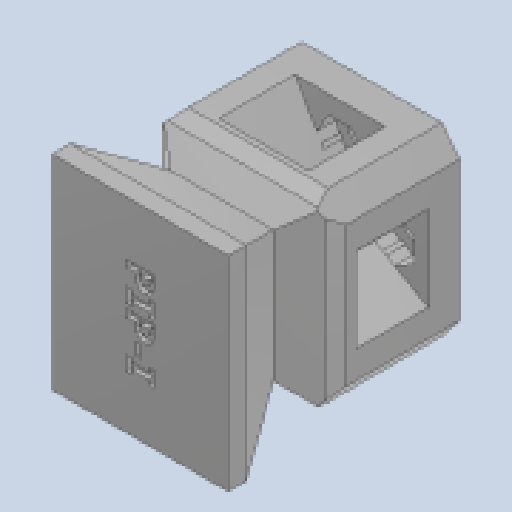
# Autodesk Inventor part: PIP-I
Saved by Autodesk Inventor 2026 (Build 300175050, 175E)
## iProperties
Created: 2025-12-11
Part Number: PIP-I
Material: Genérico
Document SubType Name: Modeling
Designer: user
Density: 1 g/cm^3
Appearance: Suave - Gris medio
Author: user
Autodesk Inventor part; units mm, degrees
ref_plane "YZ Plane" through (0, 0, 0) normal (1, 0, 0) x (0, 1, 0)
ref_plane "XZ Plane" through (0, 0, 0) normal (0, 1, 0) x (-1, 0, 0)
ref_plane "XY Plane" through (0, 0, 0) normal (0, 0, 1) x (1, 0, 0)
sketch "Boceto1" plane through (0, 0, 0) normal (0, 0, 1) x (1, 0, 0)
  line L0 (9.7, 16.5) -> (9.7, -16.5) projected
  line L1 (9.7, 16.5) -> (-9.7, 16.5) projected
  line L2 (-9.7, -16.5) -> (-9.7, 16.5) projected
  line L3 (9.7, -16.5) -> (-9.7, -16.5) projected
  circle A0 centre (8, 8) radius 0.8 construction
  circle A1 centre (-8, -8) radius 0.8 construction
  circle A2 centre (8, -8) radius 0.8 construction
  circle A3 centre (0, 0) radius 4 construction
  circle A4 centre (0, -6) radius 1.025 construction
  circle A5 centre (6, 0) radius 1.025 construction
  circle A6 centre (0, 6) radius 1.025 construction
  circle A7 centre (-6, 0) radius 1.025 construction
  circle A8 centre (-5.6569, -5.6569) radius 1.025 construction
  circle A9 centre (5.6569, -5.6569) radius 1.025 construction
  circle A10 centre (-5.6569, 5.6569) radius 1.025 construction
  circle A11 centre (5.6569, 5.6569) radius 1.025 construction
  circle A12 centre (3, 9) radius 1.025 construction
  circle A13 centre (-3, 9) radius 1.025 construction
  circle A14 centre (3, -9) radius 1.025 construction
  circle A15 centre (-3, -9) radius 1.025 construction
  circle A16 centre (6, 12) radius 1.025 construction
  circle A17 centre (0, 12) radius 1.025 construction
  circle A18 centre (-6, 12) radius 1.025 construction
  circle A19 centre (6, -12) radius 1.025 construction
  circle A20 centre (0, -12) radius 1.025 construction
  circle A21 centre (-6, -12) radius 1.025 construction
  circle A22 centre (-8, 8) radius 0.8 construction
  line L4 (-4, 1.1547) -> (-3.8297, 1.1547) construction
  arc A23 (-3.8297, 1.1547) -> (-3.8297, -1.1547) centre (0, 0) ccw construction
  line L5 (-3.8297, -1.1547) -> (-4, -1.1547) construction
  line L6 (-4, -1.1547) -> (-4.7835, -1.6071) construction
  line L7 (-4.7835, -1.6071) -> (-4.8435, -1.5031) construction
  line L8 (-4.8435, -1.5031) -> (-5.2765, -1.7531) construction
  line L9 (-5.2765, -1.7531) -> (-5.2165, -1.8571) construction
  line L10 (-5.2165, -1.8571) -> (-6, -2.3094) construction
  line L11 (-6, -2.3094) -> (-8, -1.1547) construction
  line L12 (-8, -1.1547) -> (-8, -0.25) construction
  line L13 (-8, -0.25) -> (-7.88, -0.25) construction
  line L14 (-7.88, -0.25) -> (-7.88, 0.25) construction
  line L15 (-7.88, 0.25) -> (-8, 0.25) construction
  line L16 (-8, 0.25) -> (-8, 1.1547) construction
  line L17 (-8, 1.1547) -> (-6, 2.3094) construction
  line L18 (-6, 2.3094) -> (-5.2165, 1.8571) construction
  line L19 (-5.2165, 1.8571) -> (-5.2765, 1.7531) construction
  line L20 (-5.2765, 1.7531) -> (-4.8435, 1.5031) construction
  line L21 (-4.8435, 1.5031) -> (-4.7835, 1.6071) construction
  line L22 (-4.7835, 1.6071) -> (-4, 1.1547) construction
  circle A24 centre (-6, 0) radius 1.025 construction
  line L23 (-8, -1.1547) -> (-8, 1.1547) construction
  line L24 (-8, 1.1547) -> (-6, 2.3094) construction
  line L25 (-6, 2.3094) -> (-4, 1.1547) construction
  line L26 (-4, 1.1547) -> (-4, -1.1547) construction
  line L27 (-4, -1.1547) -> (-6, -2.3094) construction
  line L28 (-6, -2.3094) -> (-8, -1.1547) construction
  line L29 (-6, -2.5403) -> (-3.8, -1.2702)
  line L30 (-3.8, -1.2702) -> (-3.8, 1.2702)
  line L31 (-3.8, 1.2702) -> (-6, 2.5403)
  line L32 (-6, 2.5403) -> (-8.2, 1.2702)
  line L33 (-8.2, 1.2702) -> (-8.2, -1.2702)
  line L34 (-8.2, -1.2702) -> (-6, -2.5403)
  line L35 (-1.2702, -3.8) -> (-2.5403, -6)
  line L36 (1.2702, -3.8) -> (-1.2702, -3.8)
  line L37 (-2.5403, -6) -> (-1.2702, -8.2)
  line L38 (-1.2702, -8.2) -> (1.2702, -8.2)
  line L39 (1.2702, -8.2) -> (2.5403, -6)
  line L40 (2.5403, -6) -> (1.2702, -3.8)
  line L41 (3.8, -1.2702) -> (6, -2.5403)
  line L42 (3.8, 1.2702) -> (3.8, -1.2702)
  line L43 (6, -2.5403) -> (8.2, -1.2702)
  line L44 (8.2, -1.2702) -> (8.2, 1.2702)
  line L45 (8.2, 1.2702) -> (6, 2.5403)
  line L46 (6, 2.5403) -> (3.8, 1.2702)
  line L47 (1.2702, 3.8) -> (2.5403, 6)
  line L48 (-1.2702, 3.8) -> (1.2702, 3.8)
  line L49 (2.5403, 6) -> (1.2702, 8.2)
  line L50 (1.2702, 8.2) -> (-1.2702, 8.2)
  line L51 (-1.2702, 8.2) -> (-2.5403, 6)
  line L52 (-2.5403, 6) -> (-1.2702, 3.8)
  line L53 (-4.6835, -1.7803) -> (-5.1165, -2.0303)
  line L54 (-5.1165, -2.0303) -> (-5.1765, -1.9263)
  line L55 (-5.1765, -1.9263) -> (-4.7435, -1.6763)
  line L56 (-4.7435, -1.6763) -> (-4.6835, -1.7803)
  line L57 (-5.1765, 1.9263) -> (-5.1165, 2.0303)
  line L58 (-4.7435, 1.6763) -> (-5.1765, 1.9263)
  line L59 (-4.6835, 1.7803) -> (-4.7435, 1.6763)
  line L60 (-8.08, -0.25) -> (-8.2, -0.25)
  line L61 (-8.08, 0.25) -> (-8.08, -0.25)
  line L62 (-8.2, 0.25) -> (-8.08, 0.25)
  line L63 (1.6763, -4.7435) -> (1.7803, -4.6835)
  line L64 (1.9263, -5.1765) -> (1.6763, -4.7435)
  line L65 (2.0303, -5.1165) -> (1.9263, -5.1765)
  line L66 (0.25, -8.08) -> (0.25, -8.2)
  line L67 (-0.25, -8.08) -> (0.25, -8.08)
  line L68 (-0.25, -8.2) -> (-0.25, -8.08)
  line L69 (-1.7803, -4.6835) -> (-1.6763, -4.7435)
  line L70 (-1.6763, -4.7435) -> (-1.9263, -5.1765)
  line L71 (-1.9263, -5.1765) -> (-2.0303, -5.1165)
  line L72 (4.7435, 1.6763) -> (4.6835, 1.7803)
  line L73 (5.1765, 1.9263) -> (4.7435, 1.6763)
  line L74 (5.1165, 2.0303) -> (5.1765, 1.9263)
  line L75 (8.08, 0.25) -> (8.2, 0.25)
  line L76 (8.08, -0.25) -> (8.08, 0.25)
  line L77 (8.2, -0.25) -> (8.08, -0.25)
  line L78 (4.6835, -1.7803) -> (4.7435, -1.6763)
  line L79 (4.7435, -1.6763) -> (5.1765, -1.9263)
  line L80 (5.1765, -1.9263) -> (5.1165, -2.0303)
  line L81 (-1.6763, 4.7435) -> (-1.7803, 4.6835)
  line L82 (-1.9263, 5.1765) -> (-1.6763, 4.7435)
  line L83 (-2.0303, 5.1165) -> (-1.9263, 5.1765)
  line L84 (-0.25, 8.08) -> (-0.25, 8.2)
  line L85 (0.25, 8.08) -> (-0.25, 8.08)
  line L86 (0.25, 8.2) -> (0.25, 8.08)
  line L87 (1.7803, 4.6835) -> (1.6763, 4.7435)
  line L88 (1.6763, 4.7435) -> (1.9263, 5.1765)
  line L89 (1.9263, 5.1765) -> (2.0303, 5.1165)
  line L90 (-9.7, -10.2) -> (9.7, -10.2)
  line L91 (-9.7, 10.2) -> (9.7, 10.2)
  point P0 (0, 0)
  point P1 (-4.9, -1.9053)
  dimension "d0" = 0.2
  dimension "d3" = 360
  dimension "d9" = 0.12
  dimension "d10" = 0.12
  dimension "d13" = 360
  dimension "d17" = 360
  dimension "d24" = 2
  dimension "d25" = 2
  constraints: 138 end point, 6 point on line, 3 parallel, 2 midpoint, 2 perpendicular, 1 coincident, 1 collinear, 174 other
  measures "d0" distance between parallel lines of L27 L29
  measures "d9" distance of L8.end L9.end
  measures "d10" distance of L53.end L54.end
  measures "d24" distance between parallel lines of L38 L90
  measures "d25" distance between parallel lines of L91 L50
extrude "Extrusión1" add sketch "Boceto1" along normal blind 3.5 contours L0 L90 L2 L91 | L54 L55 L56 L29 | L33 L62 L61 L60 | L59 L58 L57 L31 | L69 L70 L71 L35 | L40 L65 L64 L63 | L68 L67 L66 L38 | L78 L79 L80 L41 | L46 L74 L73 L72 | L77 L76 L75 L44 | L87 L88 L89 L47 | L52 L83 L82 L81 | L86 L85 L84 L50
sketch "Boceto2" plane through (0, 0, 0) normal (0, 0, -1) x (-1, 0, 0)
  line L0 (9.7, 10.2) -> (9.7, -10.2) projected
  line L1 (-9.7, -10.2) -> (-9.7, 10.2) projected
  line L2 (-1.2702, 3.8) -> (1.2702, 3.8) projected
  line L3 (-1.7803, 4.6835) -> (-1.2702, 3.8) projected
  line L4 (-1.2702, 8.2) -> (-2.5403, 6) projected
  line L5 (-0.25, 8.2) -> (-1.2702, 8.2) projected
  line L6 (2.5403, 6) -> (1.2702, 8.2) projected
  line L7 (2.0303, 5.1165) -> (2.5403, 6) projected
  line L8 (-3.8, -1.2702) -> (-3.8, 1.2702) projected
  line L9 (-4.6835, -1.7803) -> (-3.8, -1.2702) projected
  line L10 (-8.2, -1.2702) -> (-6, -2.5403) projected
  line L11 (-8.2, -0.25) -> (-8.2, -1.2702) projected
  line L12 (-6, 2.5403) -> (-8.2, 1.2702) projected
  line L13 (-5.1165, 2.0303) -> (-6, 2.5403) projected
  line L14 (1.2702, -3.8) -> (-1.2702, -3.8) projected
  line L15 (1.7803, -4.6835) -> (1.2702, -3.8) projected
  line L16 (1.2702, -8.2) -> (2.5403, -6) projected
  line L17 (0.25, -8.2) -> (1.2702, -8.2) projected
  line L18 (-2.5403, -6) -> (-1.2702, -8.2) projected
  line L19 (-2.0303, -5.1165) -> (-2.5403, -6) projected
  line L20 (6, -2.5403) -> (8.2, -1.2702) projected
  line L21 (5.1165, -2.0303) -> (6, -2.5403) projected
  line L22 (3.8, 1.2702) -> (3.8, -1.2702) projected
  line L23 (4.6835, 1.7803) -> (3.8, 1.2702) projected
  line L24 (8.2, 1.2702) -> (6, 2.5403) projected
  line L25 (8.2, 0.25) -> (8.2, 1.2702) projected
  circle A0 centre (6, 0) radius 1.025 projected
  circle A1 centre (0, 6) radius 1.025 projected
  circle A2 centre (-6, 0) radius 1.025 projected
  circle A3 centre (0, -6) radius 1.025 projected
  line L26 (-1.6763, 4.7435) -> (-1.7803, 4.6835) projected
  line L27 (-1.9263, 5.1765) -> (-1.6763, 4.7435) projected
  line L28 (-2.0303, 5.1165) -> (-1.9263, 5.1765) projected
  line L29 (-2.5403, 6) -> (-2.0303, 5.1165) projected
  line L30 (-0.25, 8.08) -> (-0.25, 8.2) projected
  line L31 (0.25, 8.08) -> (-0.25, 8.08) projected
  line L32 (0.25, 8.2) -> (0.25, 8.08) projected
  line L33 (1.2702, 8.2) -> (0.25, 8.2) projected
  line L34 (1.9263, 5.1765) -> (2.0303, 5.1165) projected
  line L35 (1.6763, 4.7435) -> (1.9263, 5.1765) projected
  line L36 (1.7803, 4.6835) -> (1.6763, 4.7435) projected
  line L37 (1.2702, 3.8) -> (1.7803, 4.6835) projected
  line L38 (-4.7435, -1.6763) -> (-4.6835, -1.7803) projected
  line L39 (-5.1765, -1.9263) -> (-4.7435, -1.6763) projected
  line L40 (-5.1165, -2.0303) -> (-5.1765, -1.9263) projected
  line L41 (-6, -2.5403) -> (-5.1165, -2.0303) projected
  line L42 (-8.08, -0.25) -> (-8.2, -0.25) projected
  line L43 (-8.08, 0.25) -> (-8.08, -0.25) projected
  line L44 (-8.2, 0.25) -> (-8.08, 0.25) projected
  line L45 (-8.2, 1.2702) -> (-8.2, 0.25) projected
  line L46 (-5.1765, 1.9263) -> (-5.1165, 2.0303) projected
  line L47 (-4.7435, 1.6763) -> (-5.1765, 1.9263) projected
  line L48 (-4.6835, 1.7803) -> (-4.7435, 1.6763) projected
  line L49 (-3.8, 1.2702) -> (-4.6835, 1.7803) projected
  line L50 (1.6763, -4.7435) -> (1.7803, -4.6835) projected
  line L51 (1.9263, -5.1765) -> (1.6763, -4.7435) projected
  line L52 (2.0303, -5.1165) -> (1.9263, -5.1765) projected
  line L53 (2.5403, -6) -> (2.0303, -5.1165) projected
  line L54 (0.25, -8.08) -> (0.25, -8.2) projected
  line L55 (-0.25, -8.08) -> (0.25, -8.08) projected
  line L56 (-0.25, -8.2) -> (-0.25, -8.08) projected
  line L57 (-1.2702, -8.2) -> (-0.25, -8.2) projected
  line L58 (-1.9263, -5.1765) -> (-2.0303, -5.1165) projected
  line L59 (-1.6763, -4.7435) -> (-1.9263, -5.1765) projected
  line L60 (-1.7803, -4.6835) -> (-1.6763, -4.7435) projected
  line L61 (-1.2702, -3.8) -> (-1.7803, -4.6835) projected
  line L62 (5.1765, -1.9263) -> (5.1165, -2.0303) projected
  line L63 (4.7435, -1.6763) -> (5.1765, -1.9263) projected
  line L64 (4.6835, -1.7803) -> (4.7435, -1.6763) projected
  line L65 (3.8, -1.2702) -> (4.6835, -1.7803) projected
  line L66 (4.7435, 1.6763) -> (4.6835, 1.7803) projected
  line L67 (5.1765, 1.9263) -> (4.7435, 1.6763) projected
  line L68 (5.1165, 2.0303) -> (5.1765, 1.9263) projected
  line L69 (6, 2.5403) -> (5.1165, 2.0303) projected
  line L70 (8.08, 0.25) -> (8.2, 0.25) projected
  line L71 (8.08, -0.25) -> (8.08, 0.25) projected
  line L72 (8.2, -0.25) -> (8.08, -0.25) projected
  line L73 (8.2, -1.2702) -> (8.2, -0.25) projected
  line L74 (-9.7, 10.2) -> (9.7, 10.2) projected
  line L75 (9.7, -10.2) -> (-9.7, -10.2) projected
  point P0 (0, 0)
extrude "Extrusión2" add sketch "Boceto2" against normal blind 1.5 contours L0 L75 L1 L74 | L3 L26 L27 L28 L29 L4 L5 L30 L31 L32 L33 L6 L7 L34 L35 L36 L37 L2 | L9 L38 L39 L40 L41 L10 L11 L42 L43 L44 L45 L12 L13 L46 L47 L48 L49 L8 | L15 L50 L51 L52 L53 L16 L17 L54 L55 L56 L57 L18 L19 L58 L59 L60 L61 L14 | L21 L62 L63 L64 L65 L22 L23 L66 L67 L68 L69 L24 L25 L70 L71 L72 L73 L20
chamfer "Chaflán1" distance 0.12 distance2 2 12 edges at (4.96, 1.8013, 3.5) (8.08, 0, 3.5) (4.96, -1.8013, 3.5) (-1.8013, -4.96, 3.5) (1.8013, -4.96, 3.5) (0, -8.08, 3.5) (-1.8013, 4.96, 3.5) (1.8013, 4.96, 3.5) (0, 8.08, 3.5) (-8.08, 0, 3.5) (-4.96, -1.8013, 3.5) (-4.96, 1.8013, 3.5) measured on face at (6.0801, -6.2468, 3.5)
sketch "Boceto3" plane through (0, 0, 3.5) normal (0, 0, 1) x (0, 1, 0)
  line L0 (4.6835, -1.7803) -> (3.8, -1.2702) projected
  line L1 (3.8, -1.2702) -> (3.8, 1.2702) projected
  line L2 (3.8, 1.2702) -> (4.6835, 1.7803) projected
  line L3 (5.1165, 2.0303) -> (6, 2.5403) projected
  line L4 (6, 2.5403) -> (8.2, 1.2702) projected
  line L5 (8.2, 1.2702) -> (8.2, 0.25) projected
  line L6 (8.2, -0.25) -> (8.2, -1.2702) projected
  line L7 (8.2, -1.2702) -> (6, -2.5403) projected
  line L8 (6, -2.5403) -> (5.1165, -2.0303) projected
  line L9 (-4.6835, 1.7803) -> (-3.8, 1.2702) projected
  line L10 (-3.8, 1.2702) -> (-3.8, -1.2702) projected
  line L11 (-3.8, -1.2702) -> (-4.6835, -1.7803) projected
  line L12 (-5.1165, -2.0303) -> (-6, -2.5403) projected
  line L13 (-6, -2.5403) -> (-8.2, -1.2702) projected
  line L14 (-8.2, -1.2702) -> (-8.2, -0.25) projected
  line L15 (-8.2, 0.25) -> (-8.2, 1.2702) projected
  line L16 (-8.2, 1.2702) -> (-6, 2.5403) projected
  line L17 (-6, 2.5403) -> (-5.1165, 2.0303) projected
  line L18 (10.2, 9.7) -> (-10.2, 9.7) projected
  line L19 (-10.2, 9.7) -> (-10.2, -9.7) projected
  line L20 (-10.2, -9.7) -> (10.2, -9.7) projected
  line L21 (10.2, -9.7) -> (10.2, 9.7) projected
  line L22 (-1.7803, -4.6835) -> (-1.2702, -3.8) projected
  line L23 (-1.2702, -3.8) -> (1.2702, -3.8) projected
  line L24 (1.2702, -3.8) -> (1.7803, -4.6835) projected
  line L25 (2.0303, -5.1165) -> (2.5403, -6) projected
  line L26 (2.5403, -6) -> (1.2702, -8.2) projected
  line L27 (1.2702, -8.2) -> (0.25, -8.2) projected
  line L28 (-0.25, -8.2) -> (-1.2702, -8.2) projected
  line L29 (-1.2702, -8.2) -> (-2.5403, -6) projected
  line L30 (-2.5403, -6) -> (-2.0303, -5.1165) projected
  line L31 (-2.0303, 5.1165) -> (-2.5403, 6) projected
  line L32 (-2.5403, 6) -> (-1.2702, 8.2) projected
  line L33 (-1.2702, 8.2) -> (-0.25, 8.2) projected
  line L34 (0.25, 8.2) -> (1.2702, 8.2) projected
  line L35 (1.2702, 8.2) -> (2.5403, 6) projected
  line L36 (2.5403, 6) -> (2.0303, 5.1165) projected
  line L37 (1.7803, 4.6835) -> (1.2702, 3.8) projected
  line L38 (1.2702, 3.8) -> (-1.2702, 3.8) projected
  line L39 (-1.2702, 3.8) -> (-1.7803, 4.6835) projected
  circle A0 centre (0, 6) radius 1.025 projected
  line L40 (1.2702, 3.8) -> (-1.2702, 3.8) projected
  line L41 (-1.2702, 3.8) -> (-4.6765, 9.7)
  line L42 (1.2702, 3.8) -> (4.6765, 9.7)
  line L43 (3.8, 1.2702) -> (10.2, 4.9652)
  line L44 (3.8, -1.2702) -> (10.2, -4.9652)
  line L45 (10.2603, 5) -> (10.2, 5)
  line L46 (10.2603, -5) -> (10.2, -5)
  line L47 (-3.8, 0) -> (3.8, 0) construction
  line L48 (0, 3.8) -> (0, -3.8) construction
  line L49 (-1.2702, -3.8) -> (-4.6765, -9.7)
  line L50 (1.2702, -3.8) -> (4.6765, -9.7)
  line L51 (-3.8, 1.2702) -> (-10.2, 4.9652)
  line L52 (-3.8, -1.2702) -> (-10.2, -4.9652)
  line L53 (-10.2603, 5) -> (-10.2, 5)
  line L54 (-10.2603, -5) -> (-10.2, -5)
  line L55 (1.7803, 4.6835) -> (2.0303, 5.1165) projected
  line L56 (-2.0303, 5.1165) -> (-1.7803, 4.6835) projected
  line L57 (0.25, 8.2) -> (-0.25, 8.2) projected
  line L58 (8.2, -0.25) -> (8.2, 0.25) projected
  line L59 (4.6835, -1.7803) -> (5.1165, -2.0303) projected
  line L60 (5.1165, 2.0303) -> (4.6835, 1.7803) projected
  line L61 (-8.2, 0.25) -> (-8.2, -0.25) projected
  line L62 (-4.6835, 1.7803) -> (-5.1165, 2.0303) projected
  line L63 (-5.1165, -2.0303) -> (-4.6835, -1.7803) projected
  line L64 (-1.7803, -4.6835) -> (-2.0303, -5.1165) projected
  line L65 (2.0303, -5.1165) -> (1.7803, -4.6835) projected
  line L66 (-0.25, -8.2) -> (0.25, -8.2) projected
  point P0 (0, 0)
  point P1 (2.0509, 5.1522)
  point P2 (-11.2, 5)
  point P3 (-10.2, -5)
  point P4 (5.1616, -2.0563)
  dimension "d26" = 9.3531
  dimension "d27" = 10
  constraints: 28 end point, 10 point on line, 8 symmetric about line, 4 collinear, 4 midpoint, 1 parallel, 1 perpendicular, 1 other
  measures "d26" distance of L41.end L42.end
  measures "d27" distance between parallel lines of L46 L45
extrude "Extrusión3" add sketch "Boceto3" along normal blind 2 contours L44 L8 L21 L20 L50 L25 L24 L23 L22 L49 L30 L19 L52 L12 L11 L10 L9 L51 L17 L18 L41 L31 L39 L38 L37 L42 L36 L43 L3 L2 L1 L0
sketch "Boceto8" plane through (0, 0, 5.5) normal (0, 0, 1) x (1, 0, 0)
  line L0 (-9.7, -10.2) -> (9.7, -10.2)
  line L1 (9.7, -10.2) -> (9.7, 10.2)
  line L2 (9.7, 10.2) -> (-9.7, 10.2)
  line L3 (-9.7, 10.2) -> (-9.7, -10.2)
  point P0 (0, 0)
  constraints: 8 end point, 2 coincident, 2 parallel, 1 horizontal, 1 perpendicular
extrude "Extrusión7" add sketch "Boceto8" along normal blind 8
chamfer "Chaflán3" distance 5.9 angle 45 1 edges at (-9.7, 0, 5.5) measured on face at (-9.7, 1.5588, 10.8333)
chamfer "Chaflán4" distance 6.4 angle 45 1 edges at (0, 10.2, 5.5) measured on face at (1.6551, 10.2, 10.8333)
chamfer "Chaflán5" distance 6.4 angle 45 1 edges at (0, -10.2, 5.5) measured on face at (-1.6551, -10.2, 10.8333)
chamfer "Chaflán6" distance 5.9 angle 45 1 edges at (9.7, 0, 5.5) measured on face at (9.7, 1.5588, 10.8333)
sketch "Boceto5" plane through (0, 0, 0) normal (1, 0, 0) x (0, 1, 0)
  line L0 (0, 13.5) -> (0, 25.5) construction
  line L1 (11.2415, 23.5) -> (7.2, 16.5)
  line L2 (-10.2, 13.5) -> (10.2, 13.5) projected
  line L3 (11.2415, 23.5) -> (11.2415, 25.5)
  line L4 (11.2415, 25.5) -> (-11.2415, 25.5)
  line L5 (10.2, 0) -> (10.2, 13.5) projected
  line L6 (7.2, 16.5) -> (10.2, 13.5)
  line L7 (-11.2415, 23.5) -> (-7.2, 16.5)
  line L8 (-11.2415, 23.5) -> (-11.2415, 25.5)
  line L9 (-7.2, 16.5) -> (-10.2, 13.5)
  line L10 (10.2, 13.5) -> (-10.2, 13.5) projected
  point P0 (0, 0)
  dimension "d69" = 60
  dimension "d71" = 2
  dimension "d72" = 12
  dimension "d79" = -1.0414
  dimension "d91" = 14.4
  dimension "d92" = 3
  dimension "d94" = 0
  dimension "d98" = 45
  constraints: 18 end point, 3 symmetric about line, 2 midpoint, 2 perpendicular, 1 horizontal alignment, 1 vertical
  measures "d69" angle of L2 L1
  measures "d71" distance of L1.start L3.end
  measures "d72" distance between parallel lines of L2 L4
  measures "d79" distance between parallel lines of L5 L3
  measures "d91" distance of L7.end L1.end
  measures "d92" distance from line of L2 L1.end
  measures "d94" distance of L2.end L6.end
  measures "d98" angle of L2 L6
extrude "Extrusión5" add sketch "Boceto5" against normal up to surface (9.7 mm away)
sketch "Boceto10" plane through (0, 0, 0) normal (0, 1, 0) x (-1, 0, 0)
  line L0 (0, 25.5) -> (9.7, 25.5) projected
  line L1 (9.7, 3.5) -> (9.7, 11.4) projected
  line L2 (9.7, 3.5) -> (9.7, 11.4) projected
  line L3 (9.7, 0) -> (9.7, 13.5) projected
  line L4 (9.7, 25.5) -> (9.7, 23.5) projected
  line L5 (9.7, 23.5) -> (9.7, 25.5) projected
  line L6 (9.7, 16.5) -> (9.7, 23.5) projected
  line L7 (9.7, 0) -> (9.7, 13.5) projected
  line L8 (0, 16.5) -> (0, 23.5) projected
  line L9 (0, 23.5) -> (0, 25.5) projected
  line L10 (0, 25.5) -> (0, 23.5) projected
  line L11 (0, 13.5) -> (-9.7, 13.5) projected
  line L12 (-9.7, 13.5) -> (0, 13.5) projected
  line L13 (9.7, 23.5) -> (3.9265, 13.5)
  line L14 (0, 23.5) -> (0, 16.5) projected
  line L15 (0, 16.5) -> (0, 13.5) projected
  line L16 (0, 13.5) -> (0, 16.5) projected
  line L17 (9.7, 16.5) -> (9.7, 13.5) projected
  line L18 (9.7, 23.5) -> (9.7, 16.5) projected
  line L19 (9.7, 13.5) -> (9.7, 16.5) projected
  line L20 (9.7, 13.5) -> (5.6585, 16.5)
  line L21 (9.7, 13.5) -> (0, 13.5) projected
  line L22 (0, 16.5) -> (9.7, 16.5) construction
  point P0 (0, 0)
  point P1 (9.7, 26.5)
  point P2 (9.7, 23.5)
  dimension "d97" = 0
  dimension "d99" = 60
  dimension "d100" = 36.587
  constraints: 4 end point, 4 point on line, 1 other
  measures "d97" distance of L3.end L20.start
  measures "d99" angle of L21 L13
  measures "d100" angle of L21 L20
extrude "Extrusión8" cut sketch "Boceto10" along normal through all both and the other way through all contours L6 L17 L20 L13
mirror "Simetría1" about plane through (0, 0, 0) normal (1, 0, 0) of "Extrusión5", "Extrusión8"
chamfer "Chaflán7" distance 2 distance2 2.5 4 edges at (-9.7, -10.2, 1.75) (-9.7, -10.2, 9.5) (9.7, -10.2, 9.5) (9.7, -10.2, 1.75) measured on face at (-1.6551, -10.2, 1.1667) measured on face at (-1.6551, -10.2, 10.8333)
chamfer "Chaflán8" distance 2 distance2 2.5 3 edges at (9.7, 10.2, 9.5) (9.7, 10.2, 1.75) (-9.7, 10.2, 6.75) measured on face at (1.6551, 10.2, 1.1667)
chamfer "Chaflán2" distance 1 angle 45 4 edges at (0, 10.2, 13.5) (0, -10.2, 13.5) (-9.7, 0, 13.5) (9.7, 0, 13.5)
fillet "Empalme1" [suppressed]
sketch "Boceto11" plane through (-9.7, -11.2415, 25.5) normal (0, 0, 1) x (1, 0, 0)
  line L0 (19.4, 22.4829) -> (19.4, 0) construction
  line L1 (19.4, 0) -> (0, 0) construction
  line L2 (0, 0) -> (0, 22.4829) construction
  line L3 (0, 22.4829) -> (19.4, 22.4829) construction
  line L4 (0, 22.4829) -> (0, 0) construction
  line L5 (0, 0) -> (19.4, 0) construction
  line L6 (19.4, 22.4829) -> (19.4, 0) construction
  line L7 (0, 22.4829) -> (19.4, 22.4829) construction
  spline S0 degree 2 poles (10.2543, 14.2171) (10.0452, 14.2171) (9.666, 14.3509) (9.5395, 14.4748) knots 0 0 0 1 2 2 2
  spline S1 degree 2 poles (9.5395, 14.4748) (9.4593, 14.5502) (9.328, 14.735) (9.2818, 14.8444) knots 0 0 0 1 2 2 2
  spline S2 degree 2 poles (9.2818, 14.8444) (9.2357, 14.9562) (9.1822, 15.2163) (9.1822, 15.3768) knots 0 0 0 1 2 2 2
  line L8 (9.1822, 15.3768) -> (9.1822, 15.7706)
  line L9 (9.1822, 15.7706) -> (8.2, 15.7706)
  line L10 (8.2, 15.7706) -> (8.2, 16.5243)
  line L11 (8.2, 16.5243) -> (11.2, 16.5243)
  line L12 (11.2, 16.5243) -> (11.2, 15.3598)
  spline S3 degree 2 poles (11.2, 15.3598) (11.2, 15.1021) (11.1052, 14.7252) (11.0031, 14.5721) knots 0 0 0 1 2 2 2
  spline S4 degree 2 poles (11.0031, 14.5721) (10.8888, 14.4019) (10.5144, 14.2171) (10.2543, 14.2171) knots 0 0 0 1 2 2 2
  spline S5 degree 2 poles (10.2348, 14.9902) (10.3637, 14.9902) (10.546, 15.1118) (10.5801, 15.1945) knots 0 0 0 1 2 2 2
  spline S6 degree 2 poles (10.5801, 15.1945) (10.6263, 15.3014) (10.6408, 15.4959) (10.6408, 15.6637) knots 0 0 0 1 2 2 2
  line L13 (10.6408, 15.6637) -> (10.6408, 15.7706)
  line L14 (10.6408, 15.7706) -> (9.7413, 15.7706)
  line L15 (9.7413, 15.7706) -> (9.7413, 15.7171)
  spline S7 degree 2 poles (9.7413, 15.7171) (9.7413, 15.6126) (9.7462, 15.423) (9.7583, 15.3525) knots 0 0 0 1 2 2 2
  spline S8 degree 2 poles (9.7583, 15.3525) (9.7681, 15.2917) (9.8264, 15.158) (9.8629, 15.1215) knots 0 0 0 1 2 2 2
  spline S9 degree 2 poles (9.8629, 15.1215) (9.9358, 15.0437) (10.0987, 14.9902) (10.2348, 14.9902) knots 0 0 0 1 2 2 2
  line L16 (8.2, 12.3209) -> (8.2, 13.9351)
  line L17 (8.2, 13.9351) -> (8.7227, 13.9351)
  line L18 (8.7227, 13.9351) -> (8.7227, 13.5048)
  line L19 (8.7227, 13.5048) -> (10.6773, 13.5048)
  line L20 (10.6773, 13.5048) -> (10.6773, 13.9351)
  line L21 (10.6773, 13.9351) -> (11.2, 13.9351)
  line L22 (11.2, 13.9351) -> (11.2, 12.3209)
  line L23 (11.2, 12.3209) -> (10.6773, 12.3209)
  line L24 (10.6773, 12.3209) -> (10.6773, 12.7512)
  line L25 (10.6773, 12.7512) -> (8.7227, 12.7512)
  line L26 (8.7227, 12.7512) -> (8.7227, 12.3209)
  line L27 (8.7227, 12.3209) -> (8.2, 12.3209)
  spline S10 degree 2 poles (10.2543, 9.5129) (10.0452, 9.5129) (9.666, 9.6466) (9.5395, 9.7706) knots 0 0 0 1 2 2 2
  spline S11 degree 2 poles (9.5395, 9.7706) (9.4593, 9.846) (9.328, 10.0308) (9.2818, 10.1402) knots 0 0 0 1 2 2 2
  spline S12 degree 2 poles (9.2818, 10.1402) (9.2357, 10.252) (9.1822, 10.5121) (9.1822, 10.6726) knots 0 0 0 1 2 2 2
  line L28 (9.1822, 10.6726) -> (9.1822, 11.0664)
  line L29 (9.1822, 11.0664) -> (8.2, 11.0664)
  line L30 (8.2, 11.0664) -> (8.2, 11.8201)
  line L31 (8.2, 11.8201) -> (11.2, 11.8201)
  line L32 (11.2, 11.8201) -> (11.2, 10.6556)
  spline S13 degree 2 poles (11.2, 10.6556) (11.2, 10.3979) (11.1052, 10.021) (11.0031, 9.8679) knots 0 0 0 1 2 2 2
  spline S14 degree 2 poles (11.0031, 9.8679) (10.8888, 9.6977) (10.5144, 9.5129) (10.2543, 9.5129) knots 0 0 0 1 2 2 2
  spline S15 degree 2 poles (10.2348, 10.286) (10.3637, 10.286) (10.546, 10.4076) (10.5801, 10.4902) knots 0 0 0 1 2 2 2
  spline S16 degree 2 poles (10.5801, 10.4902) (10.6263, 10.5972) (10.6408, 10.7917) (10.6408, 10.9594) knots 0 0 0 1 2 2 2
  line L33 (10.6408, 10.9594) -> (10.6408, 11.0664)
  line L34 (10.6408, 11.0664) -> (9.7413, 11.0664)
  line L35 (9.7413, 11.0664) -> (9.7413, 11.0129)
  spline S17 degree 2 poles (9.7413, 11.0129) (9.7413, 10.9084) (9.7462, 10.7188) (9.7583, 10.6483) knots 0 0 0 1 2 2 2
  spline S18 degree 2 poles (9.7583, 10.6483) (9.7681, 10.5875) (9.8264, 10.4538) (9.8629, 10.4173) knots 0 0 0 1 2 2 2
  spline S19 degree 2 poles (9.8629, 10.4173) (9.9358, 10.3395) (10.0987, 10.286) (10.2348, 10.286) knots 0 0 0 1 2 2 2
  line L36 (9.2454, 7.8646) -> (9.2454, 9.1993)
  line L37 (9.2454, 9.1993) -> (9.8045, 9.1993)
  line L38 (9.8045, 9.1993) -> (9.8045, 7.8646)
  line L39 (9.8045, 7.8646) -> (9.2454, 7.8646)
  line L40 (8.2, 5.8371) -> (8.2, 7.4513)
  line L41 (8.2, 7.4513) -> (8.7227, 7.4513)
  line L42 (8.7227, 7.4513) -> (8.7227, 7.021)
  line L43 (8.7227, 7.021) -> (10.6773, 7.021)
  line L44 (10.6773, 7.021) -> (10.6773, 7.4513)
  line L45 (10.6773, 7.4513) -> (11.2, 7.4513)
  line L46 (11.2, 7.4513) -> (11.2, 5.8371)
  line L47 (11.2, 5.8371) -> (10.6773, 5.8371)
  line L48 (10.6773, 5.8371) -> (10.6773, 6.2674)
  line L49 (10.6773, 6.2674) -> (8.7227, 6.2674)
  line L50 (8.7227, 6.2674) -> (8.7227, 5.8371)
  line L51 (8.7227, 5.8371) -> (8.2, 5.8371)
  point P0 (9.7, 11.2415)
  constraints: 2 coincident, 2 other
extrude "Extrusión9" cut sketch "Boceto11" against normal blind 0.5
equation "\"d10\" = d9"
equation "\"d24\" = d25"
